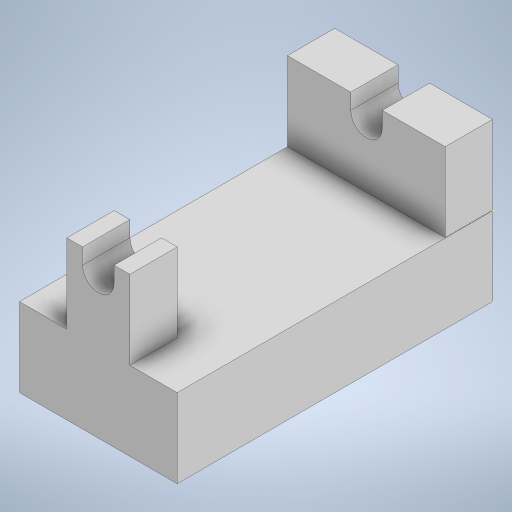
# Autodesk Inventor part: uchwyt_swiatlowod_2
Saved by Autodesk Inventor 2023 (Build 270158000, 158)
## iProperties
Created: 2022-12-19
Part Number: uchwyt_swiatlowod_2
Material: Generic
Document SubType Name: Sheet Metal
Designer: KaczorDonald
Density: 1 g/cm^3
Sheet Metal Rule: Default
Appearance: Default
Author: KaczorDonald
Autodesk Inventor part; units mm, degrees
ref_plane "YZ Plane" through (0, 0, 0) normal (1, 0, 0) x (0, 1, 0)
ref_plane "XZ Plane" through (0, 0, 0) normal (0, 1, 0) x (-1, 0, 0)
ref_plane "XY Plane" through (0, 0, 0) normal (0, 0, 1) x (1, 0, 0)
sketch "Sketch1" plane through (0, 0, 0) normal (0, 1, 0) x (-1, 0, 0)
  line L0 (0, 0) -> (10, 0)
  line L1 (10, 0) -> (10, 20)
  line L2 (10, 20) -> (0, 20)
  line L3 (0, 20) -> (0, 0)
  dimension "d0" = 10
  dimension "d1" = 20
  constraints: 8 end point, 2 parallel, 1 horizontal, 1 perpendicular
  measures "d0" distance of L2.end L1.end
  measures "d1" distance of L1.end L0.end
extrude "Extrusion1" add sketch "Sketch1" along normal blind 5
sketch "Sketch2" plane through (0, 5, 0) normal (0, 1, 0) x (1, 0, 0)
  line L0 (-10, -20) -> (0, -20) projected
  line L1 (-6.9999, -20) -> (-2.9999, -20)
  line L2 (-2.9999, -20) -> (-2.9999, -17)
  line L3 (-2.9999, -17) -> (-6.9999, -17)
  line L4 (-6.9999, -17) -> (-6.9999, -20)
  point P0 (0, 0)
  dimension "d4" = 4
  dimension "d5" = 3
  constraints: 8 end point, 2 parallel, 1 horizontal, 1 perpendicular, 1 point on line
  measures "d4" distance of L3.end L2.end
  measures "d5" distance of L2.end L1.end
extrude "Extrusion2" add sketch "Sketch2" along normal blind 5
sketch "Sketch3" plane through (0, 5, 0) normal (0, 1, 0) x (1, 0, 0)
  line L0 (-10.0114, 0) -> (-0.0114, 0)
  line L1 (-0.0114, 0) -> (-0.0114, -3)
  line L2 (-0.0114, -3) -> (-10.0114, -3)
  line L3 (-10.0114, -3) -> (-10.0114, 0)
  point P0 (0, 0)
  dimension "d8" = 10
  dimension "d9" = 3
  constraints: 8 end point, 2 parallel, 1 horizontal, 1 perpendicular
  measures "d8" distance of L1.end L2.end
  measures "d9" distance of L0.end L1.end
extrude "Extrusion3" add sketch "Sketch3" along normal blind 5
sketch "Sketch4" plane through (-10, 0, 20) normal (0, 0, 1) x (1, 0, 0)
  circle A0 centre (5.0001, 9) radius 1
  point P0 (10, 0)
  dimension "d12" = 2
  constraints: 1 centre point
  measures "d12" diameter of A0
extrude "Extrusion4" cut sketch "Sketch4" against normal blind 21.9875
sketch "Sketch5" plane through (-10, 0, 20) normal (0, 0, 1) x (1, 0, 0)
  circle A0 centre (5.0001, 9) radius 1 projected
  line L0 (4.0001, 9) -> (6.0001, 9)
  line L1 (6.0001, 9) -> (6.0001, 10)
  line L2 (6.0001, 10) -> (4.0001, 10)
  line L3 (4.0001, 10) -> (4.0001, 9)
  point P0 (10, 0)
  dimension "d15" = 2
  dimension "d16" = 1
  constraints: 8 end point, 2 parallel, 1 horizontal, 1 horizontal alignment, 1 perpendicular, 1 other
  measures "d15" distance of L2.end L1.end
  measures "d16" distance of L1.end L0.end
extrude "Extrusion5" cut sketch "Sketch5" against normal blind 22.4625 contours L3 L2 A0 | A0 L0 | A0 L2 L1 picked at (5.3251, 9.0742)
sketch "Sketch6" plane through (-10, 0, 20) normal (0, 0, 1) x (1, 0, 0)
  arc A0 (4.0001, 9) -> (6.0001, 9) centre (5.0001, 9) ccw projected
  line L0 (4.0001, 9) -> (6.0001, 9)
  line L1 (6.0001, 9) -> (6.0001, 10.3931)
  line L2 (6.0001, 10.3931) -> (4.0001, 10.3931)
  line L3 (4.0001, 10.3931) -> (4.0001, 9)
  point P0 (10, 0)
  constraints: 8 end point, 2 parallel, 1 horizontal, 1 perpendicular
extrude "Extrusion6" cut sketch "Sketch6" against normal blind 25.1625 contours L3 L2 L1 L0
sketch "Sketch7" plane through (0, 5, 0) normal (0, 1, 0) x (1, 0, 0)
  point P0 (0, 0)
sketch "Sketch8" plane through (0, 0, 0) normal (0, 0, -1) x (-1, 0, 0)
  point P0 (0, 0)
equation "\"BendRadius\" = Thickness"
equation "\"BendReliefWidth\" = Thickness"
equation "\"BendReliefDepth\" = 0.5 * Thickness"
equation "\"CornerReliefSize\" = 4 * Thickness"
equation "\"MinimumRemnant\" = 2 * Thickness"
equation "\"TransitionRadius\" = BendRadius"
equation "\"JacobiRadiusSize\" = BendRadius"
equation "\"GapSize\" = Thickness"
equation "\"Thickness\" = 3.048"
body "Solid1"
